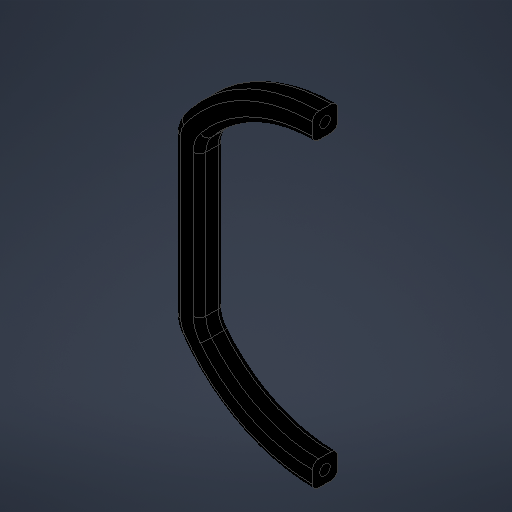
# Autodesk Inventor part: Handle
Saved by Autodesk Inventor 2026.1 (Build 301233020, 233B)
## iProperties
Created: 2025-12-04
Part Number: Handle
Material: Generic
Document SubType Name: Modeling
Designer: Bahaa
Density: 1 g/cm^3
Appearance: Default
Author: Bahaa
Autodesk Inventor part; units mm, degrees
ref_plane "YZ Plane" through (0, 0, 0) normal (1, 0, 0) x (0, 1, 0)
ref_plane "XZ Plane" through (0, 0, 0) normal (0, 1, 0) x (-1, 0, 0)
ref_plane "XY Plane" through (0, 0, 0) normal (0, 0, 1) x (1, 0, 0)
sketch "Sketch1" plane through (0, 0, 0) normal (0, 1, 0) x (-1, 0, 0)
  arc A0 (0, -60) -> (0, 60) centre (0, 0) ccw construction
  arc A1 (0, -55) -> (0, 55) centre (0, 0) ccw
  arc A2 (0, -65) -> (0, 65) centre (0, 0) ccw
  line L0 (0, 65) -> (0, 55)
  line L1 (0, -55) -> (0, -65)
  line L2 (0, 65) -> (0, -65)
  line L3 (50, 41.5331) -> (50, -41.5331)
  line L4 (45, 46.9042) -> (45, -46.9042)
  line L5 (55, 34.641) -> (55, -34.641)
  point P0 (45, 31.6228)
  point P1 (45, -31.6228)
  dimension "d16" = 60
  dimension "d17" = 5
  dimension "d18" = 5
  dimension "d19" = 10
  dimension "d20" = 10
  dimension "d21" = 0
  dimension "d25" = 5
  dimension "d26" = 5
  dimension "d27" = 55
  dimension "d28" = 55
  constraints: 12 end point, 12 point on circle, 3 centre point, 3 coincident, 3 vertical, 1 collinear, 1 parallel
  measures "d16" radius of A0
  measures "d17" radial gap between concentric circles of A1 A0
  measures "d18" radial gap between concentric circles of A0 A2
  measures "d19" distance of L1.start L1.end
  measures "d20" distance of L0.start L0.end
  measures "d21" distance from line of A0.end L0
  measures "d25" distance between parallel lines of L3 L4
  measures "d26" distance between parallel lines of L5 L3
  measures "d27" distance between parallel lines of L5 L0
  measures "d28" distance from line of A0.start L5
extrude "Extrusion1" add sketch "Sketch1" along normal blind 10 contours A1 L4 A2 L1 | L4 A1 L3 | A1 L3 A2 L4 | L0 A2 L4 A1 | L3 A1 | A1 L5 A2 L3 | L4 A2 L3 A1 | A1 L3 A2 L5
fillet "Fillet1" radius 10 2 edges at (-45, 5, -31.6228) (-45, 5, 31.6228)
fillet "Fillet2" radius 10 2 edges at (-55, 5, 34.641) (-55, 5, -34.641)
fillet "Fillet3" radius 2.5 16 edges at (-54.5346, 10, 34.6379) (-55, 10, 0) (-54.5346, 10, -34.6379) (-29.9649, 10, -57.681) (-29.9649, 10, 57.681) (-54.5346, 0, 34.6379) (-55, 0, 0) (-54.5346, 0, -34.6379) (-29.9649, 0, -57.681) (-29.9649, 0, 57.681) (-45, 10, 0) (-23.703, 10, -49.6303) (-23.703, 10, 49.6303) (-45, 0, 0) (-23.703, 0, -49.6303) (-23.703, 0, 49.6303)
sketch "Sketch2" plane through (0, 0, 62.5) normal (1, 0, 0) x (0, 0, -1)
  line L0 (7.5, 2.5) -> (7.5, 7.5) projected
  line L1 (0, 10) -> (5, 10) projected
  line L2 (-2.5, 2.5) -> (-2.5, 7.5) projected
  line L3 (0, 0) -> (5, 0) projected
  line L4 (120, 0) -> (125, 0) projected
  line L5 (127.5, 2.5) -> (127.5, 7.5) projected
  line L6 (120, 10) -> (125, 10) projected
  line L7 (117.5, 2.5) -> (117.5, 7.5) projected
  arc A0 (117.5, 2.5) -> (120, 0) centre (120, 2.5) ccw projected
  arc A1 (125, 0) -> (127.5, 2.5) centre (125, 2.5) ccw projected
  arc A2 (127.5, 7.5) -> (125, 10) centre (125, 7.5) ccw projected
  arc A3 (120, 10) -> (117.5, 7.5) centre (120, 7.5) ccw projected
  arc A4 (5, 0) -> (7.5, 2.5) centre (5, 2.5) ccw projected
  arc A5 (7.5, 7.5) -> (5, 10) centre (5, 7.5) ccw projected
  arc A6 (0, 10) -> (-2.5, 7.5) centre (0, 7.5) ccw projected
  arc A7 (-2.5, 2.5) -> (0, 0) centre (0, 2.5) ccw projected
  point P0 (122.5, 5)
  point P1 (2.5, 5)
hole "Hole1" at (0, 5, -60) at (0, 5, 60) direction (-1, 0, 0) diameter 4.2 depth 6
equation "\"d18\" = d17"
equation "\"d19\" = 2 * d17"
equation "\"d20\" = 2 * d17"
equation "\"d25\" = d17"
equation "\"d26\" = d17"
equation "\"d28\" = d27"
equation "\"d29\" = 2 * d17"
body "Solid1"
